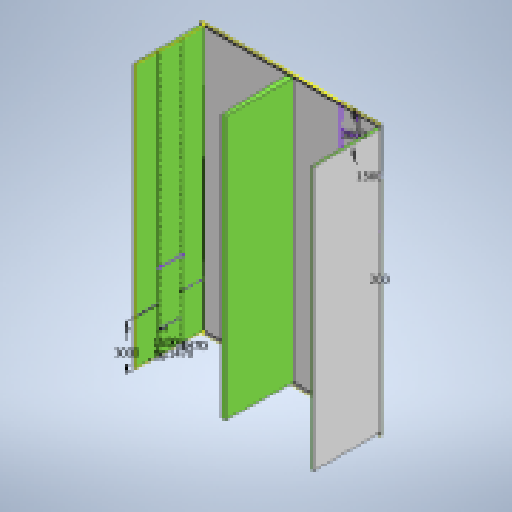
# Autodesk Inventor part: Part1
Saved by Autodesk Inventor 2026.2 (Build 302298000, 298)
## iProperties
Created: 2026-04-17
Part Number: Part1
Material: Generic
Document SubType Name: Sheet Metal
Designer: admin
Density: 1 g/cm^3
Sheet Metal Rule: Default_mm
Appearance: Default
Author: admin
Autodesk Inventor part; units mm, degrees
ref_plane "YZ Plane" through (0, 0, 0) normal (1, 0, 0) x (0, 1, 0)
ref_plane "XZ Plane" through (0, 0, 0) normal (0, 1, 0) x (-1, 0, 0)
ref_plane "XY Plane" through (0, 0, 0) normal (0, 0, 1) x (1, 0, 0)
sketch "Sketch1" plane through (0, 0, 0) normal (0, 0, 1) x (1, 0, 0)
  line L0 (6000, -9000) -> (-6000, -9000)
  line L1 (-6000, -9000) -> (-6000, 9000)
  line L2 (-6000, 9000) -> (6000, 9000)
  line L3 (6000, 9000) -> (6000, -9000)
  line L4 (6000, -9000) -> (-6000, 9000) construction
  line L5 (-6000, -9000) -> (6000, 9000) construction
  point P0 (0, 0)
  dimension "d0" = 12000
  dimension "d1" = 18000
  measures "d0" distance of L1.end L2.end
  measures "d1" distance of L0.end L1.end
extrude "Plate1" add sketch "Sketch1" along normal blind 6
sketch "Sketch2" plane through (0, 0, 6) normal (0, 0, 1) x (1, 0, 0)
  line L0 (6000, 9000) -> (6000, -9000)
  line L1 (-6000, 9000) -> (6000, 9000) projected
  line L2 (-6000, -9000) -> (-6000, 9000) projected
  line L3 (6000, -9000) -> (-6000, -9000) projected
  line L4 (5800, -8800) -> (5800, 8800)
  line L5 (5800, 8800) -> (-5800, 8800)
  line L6 (-5800, 8800) -> (-5800, -8800)
  line L7 (-5800, -8800) -> (5800, -8800)
  line L8 (6000, 9000) -> (-6000, 9000) projected
  line L9 (6000, 9000) -> (4500, 9000)
  line L10 (4500, 9000) -> (4500, 6000)
  line L11 (4500, 6000) -> (6000, 6000)
  line L12 (6000, 6000) -> (6000, 9000)
  line L13 (6000, -9000) -> (6000, 9000) projected
  line L14 (6000, 5975.1164) -> (4500, 5975.1164)
  line L15 (4500, 5975.1164) -> (4500, 2838.9347)
  line L16 (4500, 2838.9347) -> (6000, 2838.9347)
  line L17 (6000, 2838.9347) -> (6000, 5975.1164)
  line L18 (4448.9335, 7446.1559) -> (3367.2381, 7446.1559)
  line L19 (3367.2381, 7446.1559) -> (3367.2381, 4345.2957)
  line L20 (3367.2381, 4345.2957) -> (4448.9335, 4345.2957)
  line L21 (4448.9335, 4345.2957) -> (4448.9335, 7446.1559)
  line L22 (6000, 6064.0733) -> (4383.2518, 6064.0733) construction
  line L23 (4383.2518, 6064.0733) -> (4383.2518, 5895.7258) construction
  line L24 (4383.2518, 5895.7258) -> (6000, 5895.7258) construction
  line L25 (6000, 5895.7258) -> (6000, 6064.0733) construction
  line L26 (4383.2518, 5895.7258) -> (4569.2282, 5895.7258) construction
  line L27 (4569.2282, 5895.7258) -> (4569.2282, 4470.5931) construction
  line L28 (4569.2282, 4470.5931) -> (4383.2518, 4470.5931) construction
  line L29 (4383.2518, 4470.5931) -> (4383.2518, 5895.7258) construction
  line L30 (4448.9335, 9000) -> (3367.2381, 9000)
  line L31 (3367.2381, 9000) -> (3367.2381, 7500)
  line L32 (3367.2381, 7500) -> (4448.9335, 7500)
  line L33 (4448.9335, 7500) -> (4448.9335, 9000)
  line L34 (4569.2282, 7703.5758) -> (4383.2518, 7703.5758) construction
  line L35 (4383.2518, 7703.5758) -> (4383.2518, 6064.0733) construction
  line L36 (4383.2518, 6064.0733) -> (4569.2282, 6064.0733) construction
  line L37 (4569.2282, 6064.0733) -> (4569.2282, 7703.5758) construction
  dimension "d17" = 200
  dimension "d18" = 1500
  dimension "d19" = 3000
  constraints: 66 end point, 14 parallel, 7 horizontal, 7 perpendicular, 3 point on line, 3 other
  measures "d17" distance between parallel lines of L0 L4
  measures "d18" distance of L11.end L10.end
  measures "d19" distance of L10.end L9.end
sketch "Sketch4" plane through (0, 0, 0) normal (0, 1, 0) x (-1, 0, 0)
  line L0 (6000, 6) -> (-6000, 6) projected
  line L1 (-6000, 6) -> (6000, 6) projected
  line L2 (5800, 6) -> (5884.1342, 4506)
  line L3 (200, 6) -> (115.8658, 4506)
  line L4 (-115.8658, 4506) -> (-200, 6)
  line L5 (-5800, 6) -> (-5884.1342, 4506)
  line L6 (-5884.1342, 4506) -> (-6000, 4506)
  line L7 (-6000, 4506) -> (-6000, 6)
  line L8 (6000, 6) -> (6000, 4506)
  line L9 (6000, 4506) -> (5884.1342, 4506)
  line L10 (0, 0) -> (0, 4506)
  line L11 (0, 4506) -> (115.8658, 4506)
  line L12 (0, 4506) -> (-115.8658, 4506)
  point P0 (-200, 6)
  dimension "d21" = 4500
  dimension "d23" = 200
  dimension "d24" = 200
  dimension "d25" = 115.8658
  constraints: 22 end point, 4 horizontal, 4 point on line, 2 collinear, 2 equal length, 2 vertical, 1 perpendicular, 2 other
  measures "d21" distance of L1.end L8.end
  measures "d23" horizontal distance of L3.start L10.start
  measures "d24" distance of L0.start L2.start
  measures "d25" distance of L2.end L8.end
extrude "Extrusion1" add sketch "Sketch4" along normal mid plane 17576.5
sketch "Sketch5" plane through (-5800, -8788.25, 6) normal (0.9998253, 0, 0.0186932) x (0.0186932, 0, -0.9998253)
  line L0 (-3.7386, -211.75) -> (-3.7386, 0) projected
  line L1 (-4502.9523, 0) -> (-3.7386, 0) projected
  line L2 (-4502.9523, 0) -> (-4502.9523, 17576.5) projected
  line L3 (-3.7386, 17576.5) -> (-4502.9523, 17576.5) projected
  line L4 (-3.7386, 17576.5) -> (-3.7386, 17788.25) projected
  line L5 (2.2603, 17788.25) -> (-3.7386, 17788.25) projected
  line L6 (2.2603, 17788.25) -> (2.2603, -211.75) projected
  line L7 (2.2603, -211.75) -> (-3.7386, -211.75) projected
  line L8 (-2937.7397, 0) -> (-2937.7397, 17576.5)
  line L9 (-1467.7397, 0) -> (-1467.7397, 17576.5)
  line L10 (-1467.7397, 3000) -> (2.2603, 3000) construction
  line L11 (-1467.7397, 1500) -> (-2937.7397, 1500) construction
  line L12 (-2937.7397, 3000) -> (-4502.9523, 3000)
  line L13 (-1437.7397, 0) -> (-1437.7397, 17576.5) construction
  line L14 (-2907.7397, 17576.5) -> (-2907.7397, 0) construction
  line L15 (-2907.7397, 1449.1913) -> (-1437.7397, 1449.1913) construction
  line L16 (-1437.7397, 1449.1913) -> (-1437.7397, 1550.8087) construction
  line L17 (-1437.7397, 1550.8087) -> (-2907.7397, 1550.8087) construction
  line L18 (-2907.7397, 1550.8087) -> (-2907.7397, 1449.1913) construction
  line L19 (-1467.7397, 2965.3819) -> (2.2603, 2965.3819) construction
  line L20 (2.2603, 2965.3819) -> (2.2603, 3034.6181) construction
  line L21 (2.2603, 3034.6181) -> (-1467.7397, 3034.6181) construction
  line L22 (-1467.7397, 3034.6181) -> (-1467.7397, 2965.3819) construction
  line L23 (-4502.9523, 2965.3819) -> (-2907.7397, 2965.3819) construction
  line L24 (-2907.7397, 2965.3819) -> (-2907.7397, 3034.6181) construction
  line L25 (-2907.7397, 3034.6181) -> (-4502.9523, 3034.6181) construction
  line L26 (-4502.9523, 3034.6181) -> (-4502.9523, 2965.3819) construction
  line L27 (-2907.7397, 5040.7564) -> (-1437.7397, 5040.7564) construction
  line L28 (-1437.7397, 5040.7564) -> (-1437.7397, 5109.9926) construction
  line L29 (-1437.7397, 5109.9926) -> (-2907.7397, 5109.9926) construction
  line L30 (-2907.7397, 5109.9926) -> (-2907.7397, 5040.7564) construction
  line L31 (-2937.7397, 5075.3745) -> (-1467.7397, 5075.3745)
  point P0 (114.4196, 8788.25)
  point P1 (-2907.7397, 1500)
  point P2 (-1437.7397, 5075.3745)
  point P3 (-2907.7397, 5075.3745)
  dimension "d28" = 1470
  dimension "d29" = 1470
  dimension "d30" = 3000
  dimension "d31" = 1500
  dimension "d32" = 30
  dimension "d33" = 30
  constraints: 48 end point, 25 point on line, 11 perpendicular, 8 parallel, 5 midpoint, 4 horizontal, 2 collinear, 1 vertical
  measures "d28" distance between parallel lines of L6 L9
  measures "d29" distance between parallel lines of L9 L8
  measures "d30" distance between parallel lines of L1 L12
  measures "d31" distance between parallel lines of L1 L11
  measures "d32" distance between parallel lines of L8 L14
  measures "d33" distance between parallel lines of L9 L13
equation "\"d29\" = d28"
equation "\"d2\" = Thickness"
equation "\"BendRadius\" = Thickness"
equation "\"BendReliefWidth\" = Thickness"
equation "\"BendReliefDepth\" = 0.5 * Thickness"
equation "\"CornerReliefSize\" = 4 * Thickness"
equation "\"MinimumRemnant\" = 2 * Thickness"
equation "\"TransitionRadius\" = BendRadius"
equation "\"JacobiRadiusSize\" = BendRadius"
equation "\"GapSize\" = Thickness"
equation "\"Thickness\" = 6"
body "Solid1"
